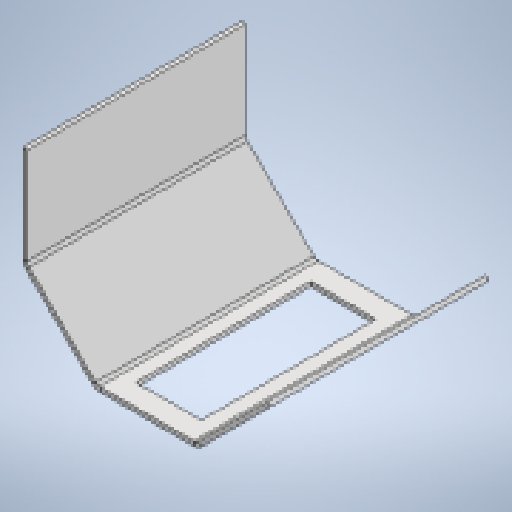
# Autodesk Inventor part: MNT-CDF-503  main tube 1
Saved by Autodesk Inventor 2025 (Build 290162010, 162A)
## iProperties
Created: 2025-01-13
Part Number: MNT-CDF-503  main tube 1
Material: Stainless Steel
Description: DIE16(5)|\ 90°|corrY -___°|X_____|bom___
Document SubType Name: Sheet Metal
Designer: user
Stock Number: МОО 305 шпангоут борт
Mass: 1762.25 g
Surface Area: 2283.33 cm^2
Volume: 220.281 cm^3
Density: 8 g/cm^3
Sheet Metal Rule: AISI304 2mm Die16
Sheet Metal Width: 0.000 mm
Sheet Metal Length: 0.000 mm
Sheet Metal Area: 0.000 mm^2
Appearance: Default
Author: user
Autodesk Inventor part; units mm, degrees
ref_plane "YZ Plane" through (0, 0, 0) normal (1, 0, 0) x (0, 1, 0)
ref_plane "XZ Plane" through (0, 0, 0) normal (0, 1, 0) x (-1, 0, 0)
ref_plane "XY Plane" through (0, 0, 0) normal (0, 0, 1) x (1, 0, 0)
sketch "Sketch1" plane through (0, 0, 0) normal (0, 0, 1) x (1, 0, 0)
  line L0 (-23.5, -50) -> (23.5, -50)
  line L1 (23.5, -50) -> (23.5, 50)
  line L2 (23.5, 50) -> (-23.5, 50)
  line L3 (-23.5, 50) -> (-23.5, -50)
  line L4 (-23.5, -50) -> (23.5, 50) construction
  line L5 (23.5, -50) -> (-23.5, 50) construction
  point P0 (0, 0)
  dimension "d154" = 47
  dimension "d155" = 100
  measures "d154" distance of L1.end L2.end
  measures "d155" distance of L0.end L1.end
extrude "Plate3" add sketch "Sketch1" along normal blind 2
sketch "Sketch7" plane through (22.0858, 50, 1.4142) normal (0.7071068, 0, -0.7071068) x (0, 1, 0)
  line L0 (-100, 0) -> (0, 0)
  line L1 (0, 0) -> (0, 47)
  line L2 (0, 47) -> (-100, 47)
  line L3 (-100, 47) -> (-100, 0)
  constraints: 6 end point, 1 horizontal, 1 perpendicular, 1 vertical
edge flange "Flange3" height 47 angle 45 thickness 2 bend radius 2.75 thickness toward (0.7071068, 0, -0.7071068) relief round relief width 2 relief depth 1 corner gap 2.75 corner form 0 edges at (23.5, 0, 2) (-23.5, 0, 2) wall of the first edge with corners at (22.0858, -50, 1.4142) (22.0858, 50, 1.4142) (55.3198, 50, 34.6482) (55.3198, -50, 34.6482)
bend "Bend3"
corner "Corner3"
sketch "Sketch8" plane through (0, 0, 2) normal (0, 0, 1) x (1, 0, 0)
  line L0 (15, 40) -> (-15, 40)
  line L1 (-15, 40) -> (-15, -20)
  line L2 (-15, -20) -> (15, -20)
  line L3 (15, -20) -> (15, 40)
  line L4 (15, 40) -> (-15, -20) construction
  line L5 (-15, 40) -> (15, -20) construction
  line L6 (-23.5, 50) -> (21.5325, 50) projected
  line L7 (-21.5325, -50) -> (21.5325, -50) projected
  line L8 (15, -50) -> (-15, -50)
  line L9 (-15, -50) -> (-15, -30)
  line L10 (-15, -30) -> (15, -30)
  line L11 (15, -30) -> (15, -50)
  point P0 (0, 0)
  point P1 (0, 10)
  point P2 (-15, -50)
  dimension "d166" = 30
  dimension "d168" = 10
  dimension "d182" = 10
  dimension "d183" = 20
  constraints: 20 end point, 4 parallel, 2 collinear, 2 horizontal, 2 midpoint, 2 perpendicular, 1 point on line, 1 vertical alignment
  measures "d166" distance of L2.end L1.end
  measures "d168" distance between parallel lines of L0 L6
  measures "d182" distance between parallel lines of L10 L2
  measures "d183" distance of L8.end L9.end
extrude "Cut1" cut sketch "Sketch8" against normal blind 2
sketch "Sketch9" plane through (-54.734, -50, 33.234) normal (-1, 0, 0) x (0, -1, 0)
  line L0 (-100, 0) -> (0, 0)
  line L1 (0, 0) -> (0, 46)
  line L2 (0, 46) -> (-100, 46)
  line L3 (-100, 46) -> (-100, 0)
  constraints: 6 end point, 1 horizontal, 1 perpendicular, 1 vertical
edge flange "Flange4" height 46 angle 45 thickness 2 bend radius 2.75 thickness toward (-1, 0, 0) relief round relief width 2 relief depth 1 edges at (-55.3198, 0, 34.6482) wall of the first edge with corners at (-54.734, 50, 33.234) (-54.734, -50, 33.234) (-54.734, -50, 79.234) (-54.734, 50, 79.234)
bend "Bend4"
corner "Corner4"
body "Solid2"
